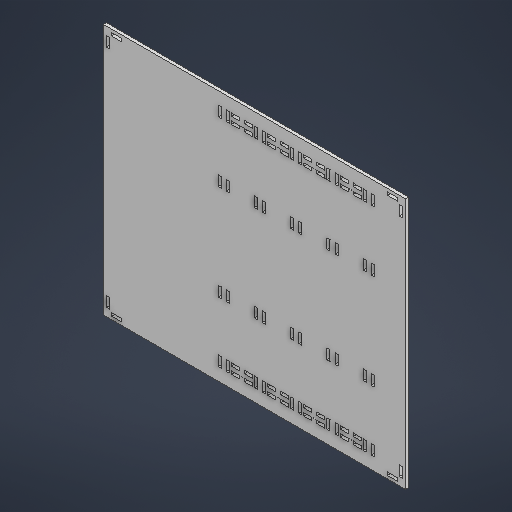
# Autodesk Inventor part: base_parqueo
Saved by Autodesk Inventor 2026 (Build 300175000, 175)
## iProperties
Created: 2026-05-15
Part Number: base_parqueo
Material: Generic
Document SubType Name: Modeling
Designer: juana
Density: 1 g/cm^3
Appearance: Default
Author: juana
Autodesk Inventor part; units mm, degrees
ref_plane "YZ Plane" through (0, 0, 0) normal (1, 0, 0) x (0, 1, 0)
ref_plane "XZ Plane" through (0, 0, 0) normal (0, 1, 0) x (-1, 0, 0)
ref_plane "XY Plane" through (0, 0, 0) normal (0, 0, 1) x (1, 0, 0)
sketch "Sketch1" plane through (0, 0, 0) normal (0, 0, 1) x (1, 0, 0)
  line L0 (300, -250) -> (0, -250)
  line L1 (0, -250) -> (0, 0)
  line L2 (0, 0) -> (300, 0)
  line L3 (300, 0) -> (300, -250)
  dimension "d0" = 250
  dimension "d1" = 300
  constraints: 8 end point, 2 coincident, 2 parallel, 1 horizontal, 1 horizontal alignment, 1 perpendicular, 1 vertical alignment
  measures "d0" distance of L2.end L0.start
  measures "d1" distance of L0.start L0.end
extrude "Extrusion1" add sketch "Sketch1" along normal blind 3
sketch "Sketch2" plane through (0, 0, 3) normal (0, 0, 1) x (1, 0, 0)
  line L0 (8, -247) -> (18, -247)
  line L1 (18, -247) -> (18, -244)
  line L2 (18, -244) -> (8, -244)
  line L3 (8, -244) -> (8, -247)
  line L4 (3, -242) -> (3, -232)
  line L5 (3, -232) -> (6, -232)
  line L6 (0, -250) -> (300, -250) construction
  line L7 (0, 0) -> (0, -250) construction
  line L8 (150, -250) -> (150, 0) construction
  line L9 (300, 0) -> (0, 0) construction
  line L10 (0, -125) -> (300, -125) construction
  line L11 (300, -250) -> (300, 0) construction
  line L12 (3, -242) -> (6, -242)
  line L13 (6, -242) -> (6, -232)
  line L14 (292, -247) -> (282, -247)
  line L15 (282, -247) -> (282, -244)
  line L16 (282, -244) -> (292, -244)
  line L17 (292, -244) -> (292, -247)
  line L18 (297, -242) -> (297, -232)
  line L19 (297, -232) -> (294, -232)
  line L20 (297, -242) -> (294, -242)
  line L21 (294, -242) -> (294, -232)
  line L22 (8, -3) -> (18, -3)
  line L23 (18, -3) -> (18, -6)
  line L24 (18, -6) -> (8, -6)
  line L25 (8, -6) -> (8, -3)
  line L26 (3, -8) -> (3, -18)
  line L27 (3, -18) -> (6, -18)
  line L28 (3, -8) -> (6, -8)
  line L29 (6, -8) -> (6, -18)
  line L30 (292, -3) -> (282, -3)
  line L31 (282, -6) -> (292, -6)
  line L32 (292, -6) -> (292, -3)
  line L33 (297, -8) -> (294, -8)
  line L34 (282, -3) -> (282, -6)
  line L35 (297, -8) -> (297, -18)
  line L36 (297, -18) -> (294, -18)
  line L37 (294, -8) -> (294, -18)
  point P0 (0, 0)
  point P1 (300, 0)
  dimension "d4" = 8
  dimension "d5" = 3
  dimension "d6" = 10
  dimension "d7" = 3
  dimension "d8" = 10
  dimension "d9" = 3
  dimension "d10" = 3
  dimension "d11" = 8
  constraints: 76 end point, 24 symmetric about line, 4 midpoint, 3 coincident, 3 horizontal, 2 parallel, 2 vertical, 1 perpendicular, 1 vertical alignment
  measures "d4" distance from line of L6.start L3
  measures "d5" distance from line of L6.start L0
  measures "d6" distance of L4.start L4.end
  measures "d7" distance of L2.end L0.start
  measures "d8" distance of L0.start L0.end
  measures "d9" distance of L4.start L12.end
  measures "d10" distance between parallel lines of L7 L4
  measures "d11" distance between parallel lines of L6 L12
extrude "Extrusion2" cut sketch "Sketch2" against normal blind 3
sketch "Sketch3" plane through (0, 0, 3) normal (0, 0, 1) x (1, 0, 0)
  line L0 (125, -12.5) -> (250, -12.5) construction
  line L1 (250, -12.5) -> (250, -237.5) construction
  line L2 (250, -237.5) -> (125, -237.5) construction
  line L3 (125, -237.5) -> (125, -12.5) construction
  line L4 (0, 0) -> (0, -250) construction
  line L5 (300, 0) -> (0, 0) construction
  line L6 (125, -12.5) -> (150, -12.5) construction
  line L7 (150, -12.5) -> (150, -82.5) construction
  line L8 (150, -82.5) -> (125, -82.5) construction
  line L9 (125, -82.5) -> (125, -12.5) construction
  line L10 (125, -12.5) -> (122, -12.5)
  line L11 (122, -12.5) -> (122, -22.5)
  line L12 (122, -22.5) -> (125, -22.5)
  line L13 (125, -22.5) -> (125, -12.5)
  line L14 (125, -82.5) -> (122, -82.5)
  line L15 (122, -82.5) -> (122, -72.5)
  line L16 (122, -72.5) -> (125, -72.5)
  line L17 (125, -72.5) -> (125, -82.5)
  line L18 (122, -72.5) -> (117, -72.5) construction
  line L19 (117, -72.5) -> (117, -82.5) construction
  line L20 (117, -82.5) -> (122, -82.5) construction
  line L21 (122, -82.5) -> (122, -72.5) construction
  line L22 (0, -125) -> (300, -125) construction
  line L23 (300, -250) -> (300, 0) construction
  line L24 (125, -47.5) -> (250, -47.5) construction
  line L25 (119.5, -72.5) -> (119.5, -82.5) construction
  line L26 (114, -82.5) -> (117, -82.5)
  line L27 (117, -82.5) -> (117, -72.5)
  line L28 (117, -72.5) -> (114, -72.5)
  line L29 (114, -72.5) -> (114, -82.5)
  line L30 (117, -82.5) -> (117, -72.5) construction
  line L31 (125, -12.5) -> (122, -12.5)
  line L32 (122, -12.5) -> (122, -22.5)
  line L33 (122, -22.5) -> (125, -22.5)
  line L34 (125, -22.5) -> (125, -12.5)
  line L35 (122, -22.5) -> (117, -22.5) construction
  line L36 (117, -22.5) -> (117, -12.5) construction
  line L37 (117, -12.5) -> (122, -12.5) construction
  line L38 (122, -12.5) -> (122, -22.5) construction
  line L39 (119.5, -22.5) -> (119.5, -12.5) construction
  line L40 (117, -22.5) -> (114, -22.5)
  line L41 (114, -22.5) -> (114, -12.5)
  line L42 (117, -12.5) -> (117, -22.5) construction
  line L43 (117, -12.5) -> (117, -22.5)
  line L44 (114, -12.5) -> (117, -12.5)
  line L45 (158, -22.5) -> (161, -22.5)
  line L46 (158, -22.5) -> (161, -22.5)
  line L47 (153, -22.5) -> (150, -22.5)
  line L48 (158, -22.5) -> (153, -22.5) construction
  line L49 (155.5, -22.5) -> (155.5, -12.5) construction
  line L50 (150, -12.5) -> (153, -12.5)
  line L51 (161, -12.5) -> (158, -12.5)
  line L52 (161, -12.5) -> (158, -12.5)
  line L53 (161, -22.5) -> (161, -12.5)
  line L54 (161, -22.5) -> (161, -12.5)
  line L55 (158, -12.5) -> (158, -22.5)
  line L56 (158, -12.5) -> (158, -22.5)
  line L57 (153, -22.5) -> (153, -12.5) construction
  line L58 (153, -12.5) -> (153, -22.5)
  line L59 (153, -12.5) -> (158, -12.5) construction
  line L60 (150, -22.5) -> (150, -12.5)
  line L61 (158, -12.5) -> (158, -22.5) construction
  line L62 (153, -12.5) -> (153, -22.5) construction
  line L63 (194, -22.5) -> (197, -22.5)
  line L64 (194, -22.5) -> (197, -22.5)
  line L65 (189, -22.5) -> (186, -22.5)
  line L66 (194, -22.5) -> (189, -22.5) construction
  line L67 (191.5, -22.5) -> (191.5, -12.5) construction
  line L68 (186, -12.5) -> (189, -12.5)
  line L69 (197, -12.5) -> (194, -12.5)
  line L70 (197, -12.5) -> (194, -12.5)
  line L71 (197, -22.5) -> (197, -12.5)
  line L72 (197, -22.5) -> (197, -12.5)
  line L73 (194, -12.5) -> (194, -22.5)
  line L74 (194, -12.5) -> (194, -22.5)
  line L75 (189, -22.5) -> (189, -12.5) construction
  line L76 (189, -12.5) -> (189, -22.5)
  line L77 (189, -12.5) -> (194, -12.5) construction
  line L78 (186, -22.5) -> (186, -12.5)
  line L79 (194, -12.5) -> (194, -22.5) construction
  line L80 (189, -12.5) -> (189, -22.5) construction
  line L81 (230, -22.5) -> (233, -22.5)
  line L82 (230, -22.5) -> (233, -22.5)
  line L83 (225, -22.5) -> (222, -22.5)
  line L84 (230, -22.5) -> (225, -22.5) construction
  line L85 (227.5, -22.5) -> (227.5, -12.5) construction
  line L86 (222, -12.5) -> (225, -12.5)
  line L87 (233, -12.5) -> (230, -12.5)
  line L88 (233, -12.5) -> (230, -12.5)
  line L89 (233, -22.5) -> (233, -12.5)
  line L90 (233, -22.5) -> (233, -12.5)
  line L91 (230, -12.5) -> (230, -22.5)
  line L92 (230, -12.5) -> (230, -22.5)
  line L93 (225, -22.5) -> (225, -12.5) construction
  line L94 (225, -12.5) -> (225, -22.5)
  line L95 (225, -12.5) -> (230, -12.5) construction
  line L96 (222, -22.5) -> (222, -12.5)
  line L97 (230, -12.5) -> (230, -22.5) construction
  line L98 (225, -12.5) -> (225, -22.5) construction
  line L99 (266, -22.5) -> (269, -22.5)
  line L100 (266, -22.5) -> (269, -22.5)
  line L101 (261, -22.5) -> (258, -22.5)
  line L102 (266, -22.5) -> (261, -22.5) construction
  line L103 (263.5, -22.5) -> (263.5, -12.5) construction
  line L104 (258, -12.5) -> (261, -12.5)
  line L105 (269, -12.5) -> (266, -12.5)
  line L106 (269, -12.5) -> (266, -12.5)
  line L107 (269, -22.5) -> (269, -12.5)
  line L108 (269, -22.5) -> (269, -12.5)
  line L109 (266, -12.5) -> (266, -22.5)
  line L110 (266, -12.5) -> (266, -22.5)
  line L111 (261, -22.5) -> (261, -12.5) construction
  line L112 (261, -12.5) -> (261, -22.5)
  line L113 (261, -12.5) -> (266, -12.5) construction
  line L114 (258, -22.5) -> (258, -12.5)
  line L115 (266, -12.5) -> (266, -22.5) construction
  line L116 (261, -12.5) -> (261, -22.5) construction
  line L117 (125, -82.5) -> (250, -82.5) construction
  line L118 (158, -72.5) -> (161, -72.5)
  line L119 (158, -72.5) -> (161, -72.5)
  line L120 (153, -72.5) -> (150, -72.5)
  line L121 (158, -72.5) -> (153, -72.5) construction
  line L122 (155.5, -72.5) -> (155.5, -82.5) construction
  line L123 (150, -82.5) -> (153, -82.5)
  line L124 (161, -82.5) -> (158, -82.5)
  line L125 (161, -82.5) -> (158, -82.5)
  line L126 (161, -72.5) -> (161, -82.5)
  line L127 (161, -72.5) -> (161, -82.5)
  line L128 (158, -82.5) -> (158, -72.5)
  line L129 (158, -82.5) -> (158, -72.5)
  line L130 (153, -72.5) -> (153, -82.5) construction
  line L131 (153, -82.5) -> (153, -72.5)
  line L132 (153, -82.5) -> (158, -82.5) construction
  line L133 (150, -72.5) -> (150, -82.5)
  line L134 (158, -82.5) -> (158, -72.5) construction
  line L135 (153, -82.5) -> (153, -72.5) construction
  line L136 (194, -72.5) -> (197, -72.5)
  line L137 (194, -72.5) -> (197, -72.5)
  line L138 (189, -72.5) -> (186, -72.5)
  line L139 (194, -72.5) -> (189, -72.5) construction
  line L140 (191.5, -72.5) -> (191.5, -82.5) construction
  line L141 (186, -82.5) -> (189, -82.5)
  line L142 (197, -82.5) -> (194, -82.5)
  line L143 (197, -82.5) -> (194, -82.5)
  line L144 (197, -72.5) -> (197, -82.5)
  line L145 (197, -72.5) -> (197, -82.5)
  line L146 (194, -82.5) -> (194, -72.5)
  line L147 (194, -82.5) -> (194, -72.5)
  line L148 (189, -72.5) -> (189, -82.5) construction
  line L149 (189, -82.5) -> (189, -72.5)
  line L150 (189, -82.5) -> (194, -82.5) construction
  line L151 (186, -72.5) -> (186, -82.5)
  line L152 (194, -82.5) -> (194, -72.5) construction
  line L153 (189, -82.5) -> (189, -72.5) construction
  line L154 (230, -72.5) -> (233, -72.5)
  line L155 (230, -72.5) -> (233, -72.5)
  line L156 (225, -72.5) -> (222, -72.5)
  line L157 (230, -72.5) -> (225, -72.5) construction
  line L158 (227.5, -72.5) -> (227.5, -82.5) construction
  line L159 (222, -82.5) -> (225, -82.5)
  line L160 (233, -82.5) -> (230, -82.5)
  line L161 (233, -82.5) -> (230, -82.5)
  line L162 (233, -72.5) -> (233, -82.5)
  line L163 (233, -72.5) -> (233, -82.5)
  line L164 (230, -82.5) -> (230, -72.5)
  line L165 (230, -82.5) -> (230, -72.5)
  line L166 (225, -72.5) -> (225, -82.5) construction
  line L167 (225, -82.5) -> (225, -72.5)
  line L168 (225, -82.5) -> (230, -82.5) construction
  line L169 (222, -72.5) -> (222, -82.5)
  line L170 (230, -82.5) -> (230, -72.5) construction
  line L171 (225, -82.5) -> (225, -72.5) construction
  line L172 (266, -72.5) -> (269, -72.5)
  line L173 (266, -72.5) -> (269, -72.5)
  line L174 (261, -72.5) -> (258, -72.5)
  line L175 (266, -72.5) -> (261, -72.5) construction
  line L176 (263.5, -72.5) -> (263.5, -82.5) construction
  line L177 (258, -82.5) -> (261, -82.5)
  line L178 (269, -82.5) -> (266, -82.5)
  line L179 (269, -82.5) -> (266, -82.5)
  line L180 (269, -72.5) -> (269, -82.5)
  line L181 (269, -72.5) -> (269, -82.5)
  line L182 (266, -82.5) -> (266, -72.5)
  line L183 (266, -82.5) -> (266, -72.5)
  line L184 (261, -72.5) -> (261, -82.5) construction
  line L185 (261, -82.5) -> (261, -72.5)
  line L186 (261, -82.5) -> (266, -82.5) construction
  line L187 (258, -72.5) -> (258, -82.5)
  line L188 (266, -82.5) -> (266, -72.5) construction
  line L189 (261, -82.5) -> (261, -72.5) construction
  line L190 (125, -237.5) -> (250, -237.5) construction
  line L191 (125, -237.5) -> (150, -237.5) construction
  line L192 (150, -237.5) -> (150, -167.5) construction
  line L193 (150, -167.5) -> (125, -167.5) construction
  line L194 (125, -167.5) -> (125, -237.5) construction
  line L195 (125, -237.5) -> (122, -237.5)
  line L196 (122, -237.5) -> (122, -227.5)
  line L197 (122, -227.5) -> (125, -227.5)
  line L198 (125, -227.5) -> (125, -237.5)
  line L199 (125, -167.5) -> (122, -167.5)
  line L200 (122, -167.5) -> (122, -177.5)
  line L201 (122, -177.5) -> (125, -177.5)
  line L202 (125, -177.5) -> (125, -167.5)
  line L203 (122, -177.5) -> (117, -177.5) construction
  line L204 (117, -177.5) -> (117, -167.5) construction
  line L205 (117, -167.5) -> (122, -167.5) construction
  line L206 (122, -167.5) -> (122, -177.5) construction
  line L207 (125, -202.5) -> (250, -202.5) construction
  line L208 (119.5, -177.5) -> (119.5, -167.5) construction
  line L209 (117, -177.5) -> (114, -177.5)
  line L210 (114, -177.5) -> (114, -167.5)
  line L211 (117, -167.5) -> (117, -177.5) construction
  line L212 (117, -167.5) -> (117, -177.5)
  line L213 (114, -167.5) -> (117, -167.5)
  line L214 (117, -227.5) -> (117, -237.5) construction
  line L215 (117, -237.5) -> (117, -227.5)
  line L216 (119.5, -227.5) -> (119.5, -237.5) construction
  line L217 (122, -237.5) -> (122, -227.5) construction
  line L218 (122, -237.5) -> (122, -227.5)
  line L219 (125, -227.5) -> (125, -237.5)
  line L220 (125, -237.5) -> (122, -237.5)
  line L221 (114, -237.5) -> (117, -237.5)
  line L222 (114, -227.5) -> (114, -237.5)
  line L223 (117, -237.5) -> (117, -227.5) construction
  line L224 (122, -227.5) -> (117, -227.5) construction
  line L225 (122, -227.5) -> (125, -227.5)
  line L226 (117, -227.5) -> (114, -227.5)
  line L227 (117, -237.5) -> (122, -237.5) construction
  line L228 (158, -227.5) -> (161, -227.5)
  line L229 (158, -227.5) -> (161, -227.5)
  line L230 (153, -227.5) -> (150, -227.5)
  line L231 (158, -227.5) -> (153, -227.5) construction
  line L232 (155.5, -227.5) -> (155.5, -237.5) construction
  line L233 (150, -237.5) -> (153, -237.5)
  line L234 (161, -237.5) -> (158, -237.5)
  line L235 (161, -237.5) -> (158, -237.5)
  line L236 (161, -227.5) -> (161, -237.5)
  line L237 (161, -227.5) -> (161, -237.5)
  line L238 (158, -237.5) -> (158, -227.5)
  line L239 (158, -237.5) -> (158, -227.5)
  line L240 (153, -227.5) -> (153, -237.5) construction
  line L241 (153, -237.5) -> (153, -227.5)
  line L242 (153, -237.5) -> (158, -237.5) construction
  line L243 (150, -227.5) -> (150, -237.5)
  line L244 (158, -237.5) -> (158, -227.5) construction
  line L245 (153, -237.5) -> (153, -227.5) construction
  line L246 (194, -227.5) -> (197, -227.5)
  line L247 (194, -227.5) -> (197, -227.5)
  line L248 (189, -227.5) -> (186, -227.5)
  line L249 (194, -227.5) -> (189, -227.5) construction
  line L250 (191.5, -227.5) -> (191.5, -237.5) construction
  line L251 (186, -237.5) -> (189, -237.5)
  line L252 (197, -237.5) -> (194, -237.5)
  line L253 (197, -237.5) -> (194, -237.5)
  line L254 (197, -227.5) -> (197, -237.5)
  line L255 (197, -227.5) -> (197, -237.5)
  line L256 (194, -237.5) -> (194, -227.5)
  line L257 (194, -237.5) -> (194, -227.5)
  line L258 (189, -227.5) -> (189, -237.5) construction
  line L259 (189, -237.5) -> (189, -227.5)
  line L260 (189, -237.5) -> (194, -237.5) construction
  line L261 (186, -227.5) -> (186, -237.5)
  line L262 (194, -237.5) -> (194, -227.5) construction
  line L263 (189, -237.5) -> (189, -227.5) construction
  line L264 (230, -227.5) -> (233, -227.5)
  line L265 (230, -227.5) -> (233, -227.5)
  line L266 (225, -227.5) -> (222, -227.5)
  line L267 (230, -227.5) -> (225, -227.5) construction
  line L268 (227.5, -227.5) -> (227.5, -237.5) construction
  line L269 (222, -237.5) -> (225, -237.5)
  line L270 (233, -237.5) -> (230, -237.5)
  line L271 (233, -237.5) -> (230, -237.5)
  line L272 (233, -227.5) -> (233, -237.5)
  line L273 (233, -227.5) -> (233, -237.5)
  line L274 (230, -237.5) -> (230, -227.5)
  line L275 (230, -237.5) -> (230, -227.5)
  line L276 (225, -227.5) -> (225, -237.5) construction
  line L277 (225, -237.5) -> (225, -227.5)
  line L278 (225, -237.5) -> (230, -237.5) construction
  line L279 (222, -227.5) -> (222, -237.5)
  line L280 (230, -237.5) -> (230, -227.5) construction
  line L281 (225, -237.5) -> (225, -227.5) construction
  line L282 (266, -227.5) -> (269, -227.5)
  line L283 (266, -227.5) -> (269, -227.5)
  line L284 (261, -227.5) -> (258, -227.5)
  line L285 (266, -227.5) -> (261, -227.5) construction
  line L286 (263.5, -227.5) -> (263.5, -237.5) construction
  line L287 (258, -237.5) -> (261, -237.5)
  line L288 (269, -237.5) -> (266, -237.5)
  line L289 (269, -237.5) -> (266, -237.5)
  line L290 (269, -227.5) -> (269, -237.5)
  line L291 (269, -227.5) -> (269, -237.5)
  line L292 (266, -237.5) -> (266, -227.5)
  line L293 (266, -237.5) -> (266, -227.5)
  line L294 (261, -227.5) -> (261, -237.5) construction
  line L295 (261, -237.5) -> (261, -227.5)
  line L296 (261, -237.5) -> (266, -237.5) construction
  line L297 (258, -227.5) -> (258, -237.5)
  line L298 (266, -237.5) -> (266, -227.5) construction
  line L299 (261, -237.5) -> (261, -227.5) construction
  line L300 (158, -177.5) -> (161, -177.5)
  line L301 (158, -177.5) -> (161, -177.5)
  line L302 (150, -177.5) -> (150, -167.5)
  line L303 (150, -167.5) -> (153, -167.5)
  line L304 (153, -177.5) -> (150, -177.5)
  line L305 (153, -167.5) -> (153, -177.5) construction
  line L306 (153, -177.5) -> (153, -167.5) construction
  line L307 (153, -167.5) -> (153, -177.5)
  line L308 (153, -167.5) -> (158, -167.5) construction
  line L309 (158, -177.5) -> (153, -177.5) construction
  line L310 (158, -167.5) -> (158, -177.5)
  line L311 (158, -167.5) -> (158, -177.5) construction
  line L312 (158, -167.5) -> (158, -177.5)
  line L313 (161, -167.5) -> (158, -167.5)
  line L314 (161, -167.5) -> (158, -167.5)
  line L315 (161, -177.5) -> (161, -167.5)
  line L316 (161, -177.5) -> (161, -167.5)
  line L317 (155.5, -177.5) -> (155.5, -167.5) construction
  line L318 (125, -167.5) -> (250, -167.5) construction
  line L319 (186, -177.5) -> (186, -167.5)
  line L320 (186, -167.5) -> (189, -167.5)
  line L321 (189, -177.5) -> (186, -177.5)
  line L322 (189, -167.5) -> (189, -177.5) construction
  line L323 (189, -177.5) -> (189, -167.5) construction
  line L324 (189, -167.5) -> (189, -177.5)
  line L325 (191.5, -177.5) -> (191.5, -167.5) construction
  line L326 (189, -167.5) -> (194, -167.5) construction
  line L327 (194, -177.5) -> (189, -177.5) construction
  line L328 (194, -167.5) -> (194, -177.5)
  line L329 (194, -167.5) -> (194, -177.5)
  line L330 (194, -177.5) -> (197, -177.5)
  line L331 (194, -177.5) -> (197, -177.5)
  line L332 (197, -167.5) -> (194, -167.5)
  line L333 (197, -167.5) -> (194, -167.5)
  line L334 (197, -177.5) -> (197, -167.5)
  line L335 (197, -177.5) -> (197, -167.5)
  line L336 (194, -167.5) -> (194, -177.5) construction
  line L337 (222, -177.5) -> (222, -167.5)
  line L338 (222, -167.5) -> (225, -167.5)
  line L339 (225, -177.5) -> (222, -177.5)
  line L340 (225, -177.5) -> (225, -167.5) construction
  line L341 (225, -167.5) -> (225, -177.5)
  line L342 (225, -167.5) -> (225, -177.5) construction
  line L343 (227.5, -177.5) -> (227.5, -167.5) construction
  line L344 (225, -167.5) -> (230, -167.5) construction
  line L345 (230, -177.5) -> (225, -177.5) construction
  line L346 (230, -167.5) -> (230, -177.5)
  line L347 (230, -167.5) -> (230, -177.5) construction
  line L348 (230, -167.5) -> (230, -177.5)
  line L349 (233, -177.5) -> (233, -167.5)
  line L350 (233, -177.5) -> (233, -167.5)
  line L351 (230, -177.5) -> (233, -177.5)
  line L352 (230, -177.5) -> (233, -177.5)
  line L353 (233, -167.5) -> (230, -167.5)
  line L354 (233, -167.5) -> (230, -167.5)
  line L355 (261, -167.5) -> (261, -177.5) construction
  line L356 (261, -177.5) -> (261, -167.5) construction
  line L357 (261, -167.5) -> (261, -177.5)
  line L358 (266, -177.5) -> (261, -177.5) construction
  line L359 (266, -167.5) -> (266, -177.5)
  line L360 (266, -167.5) -> (266, -177.5) construction
  line L361 (266, -167.5) -> (266, -177.5)
  line L362 (266, -177.5) -> (269, -177.5)
  line L363 (266, -177.5) -> (269, -177.5)
  line L364 (263.5, -177.5) -> (263.5, -167.5) construction
  line L365 (261, -177.5) -> (258, -177.5)
  line L366 (258, -177.5) -> (258, -167.5)
  line L367 (269, -177.5) -> (269, -167.5)
  line L368 (269, -177.5) -> (269, -167.5)
  line L369 (269, -167.5) -> (266, -167.5)
  line L370 (269, -167.5) -> (266, -167.5)
  line L371 (261, -167.5) -> (266, -167.5) construction
  line L372 (258, -167.5) -> (261, -167.5)
  point P0 (125, -125)
  point P1 (187.5, -12.5)
  point P2 (187.5, -82.5)
  point P3 (150, -82.5)
  point P4 (187.5, -237.5)
  point P5 (150, -167.5)
  point P6 (187.5, -167.5)
  dimension "d14" = 25
  dimension "d15" = 70
  dimension "d16" = 125
  dimension "d17" = 225
  dimension "d18" = 3
  dimension "d19" = 10
  dimension "d20" = 3
  dimension "d21" = 10
  dimension "d22" = 5
  dimension "d25" = 36
  dimension "d30" = 125
  constraints: 740 end point, 235 symmetric about line, 10 parallel, 7 horizontal, 7 midpoint, 5 perpendicular, 2 horizontal alignment, 1 coincident, 1 point on line, 1 vertical alignment, 132 other
  measures "d14" distance of L6.start L6.end
  measures "d15" distance of L6.end L7.end
  measures "d16" distance of L0.start L0.end
  measures "d17" distance of L2.end L0.start
  measures "d18" distance of L6.start L10.end
  measures "d19" distance of L10.end L11.end
  measures "d20" distance of L8.end L14.end
  measures "d21" distance of L14.end L15.end
  measures "d22" distance of L15.end L18.end
  measures "d25" distance of L0.start L52.start
  measures "d30" distance between parallel lines of L4 L3
extrude "Extrusion3" cut sketch "Sketch3" against normal blind 3
sketch "Sketch4" plane through (0, 0, 3) normal (0, 0, 1) x (1, 0, 0)
  line L0 (114, -12.5) -> (114, -22.5) construction
  line L1 (266, -237.5) -> (269, -237.5) construction
  line L2 (114, -12.5) -> (269, -12.5) construction
  line L3 (269, -12.5) -> (269, -237.5) construction
  line L4 (269, -237.5) -> (114, -237.5) construction
  line L5 (114, -237.5) -> (114, -12.5) construction
  line L6 (114, -167.5) -> (117, -167.5) construction
  line L7 (125, -177.5) -> (125, -167.5) construction
  line L8 (114, -167.5) -> (125, -167.5) construction
  line L9 (125, -167.5) -> (125, -177.5) construction
  line L10 (125, -177.5) -> (114, -177.5) construction
  line L11 (114, -177.5) -> (114, -167.5) construction
  line L12 (114, -227.5) -> (125, -227.5) construction
  line L13 (125, -227.5) -> (125, -237.5) construction
  line L14 (125, -237.5) -> (114, -237.5) construction
  line L15 (114, -237.5) -> (114, -227.5) construction
  line L16 (127, -227.5) -> (135, -227.5)
  line L17 (135, -227.5) -> (135, -230.5)
  line L18 (135, -230.5) -> (127, -230.5)
  line L19 (127, -230.5) -> (127, -227.5)
  line L20 (114, -227.5) -> (161, -227.5) construction
  line L21 (161, -227.5) -> (161, -237.5) construction
  line L22 (161, -237.5) -> (114, -237.5) construction
  line L23 (114, -237.5) -> (114, -227.5) construction
  line L24 (137.5, -227.5) -> (137.5, -237.5) construction
  line L25 (148, -227.5) -> (140, -227.5)
  line L26 (140, -227.5) -> (140, -230.5)
  line L27 (140, -230.5) -> (148, -230.5)
  line L28 (148, -230.5) -> (148, -227.5)
  circle A0 centre (137.5, -230.65) radius 0.15
  circle A1 centre (138.5, -230.65) radius 0.15
  circle A2 centre (136.5, -230.65) radius 0.15
  line L29 (140, -230.5) -> (134.9519, -230.5) construction
  line L30 (125, -232.5) -> (150, -232.5) construction
  line L31 (150, -227.5) -> (150, -237.5) construction
  line L32 (127, -237.5) -> (135, -237.5)
  line L33 (135, -237.5) -> (135, -234.5)
  line L34 (135, -234.5) -> (127, -234.5)
  line L35 (127, -234.5) -> (127, -237.5)
  line L36 (148, -237.5) -> (140, -237.5)
  line L37 (140, -237.5) -> (140, -234.5)
  line L38 (140, -234.5) -> (148, -234.5)
  line L39 (148, -234.5) -> (148, -237.5)
  circle A3 centre (137.5, -234.35) radius 0.15
  circle A4 centre (138.5, -234.35) radius 0.15
  circle A5 centre (136.5, -234.35) radius 0.15
  line L40 (140, -234.5) -> (134.9519, -234.5) construction
  line L41 (171, -230.5) -> (163, -230.5)
  line L42 (171, -227.5) -> (171, -230.5)
  line L43 (176, -230.5) -> (170.9519, -230.5) construction
  circle A6 centre (172.5, -230.65) radius 0.15
  circle A7 centre (173.5, -230.65) radius 0.15
  circle A8 centre (174.5, -230.65) radius 0.15
  circle A9 centre (172.5, -234.35) radius 0.15
  circle A10 centre (173.5, -234.35) radius 0.15
  circle A11 centre (174.5, -234.35) radius 0.15
  line L44 (173.5, -227.5) -> (173.5, -237.5) construction
  line L45 (163, -237.5) -> (171, -237.5)
  line L46 (171, -237.5) -> (171, -234.5)
  line L47 (171, -234.5) -> (163, -234.5)
  line L48 (163, -227.5) -> (171, -227.5)
  line L49 (163, -234.5) -> (163, -237.5)
  line L50 (176, -234.5) -> (170.9519, -234.5) construction
  line L51 (163, -230.5) -> (163, -227.5)
  line L52 (184, -227.5) -> (176, -227.5)
  line L53 (176, -227.5) -> (176, -230.5)
  line L54 (176, -230.5) -> (184, -230.5)
  line L55 (184, -230.5) -> (184, -227.5)
  line L56 (176, -237.5) -> (176, -234.5)
  line L57 (184, -237.5) -> (176, -237.5)
  line L58 (176, -234.5) -> (184, -234.5)
  line L59 (184, -234.5) -> (184, -237.5)
  line L60 (207, -230.5) -> (199, -230.5)
  line L61 (207, -227.5) -> (207, -230.5)
  line L62 (212, -230.5) -> (206.9519, -230.5) construction
  circle A12 centre (208.5, -230.65) radius 0.15
  circle A13 centre (209.5, -230.65) radius 0.15
  circle A14 centre (210.5, -230.65) radius 0.15
  circle A15 centre (208.5, -234.35) radius 0.15
  circle A16 centre (209.5, -234.35) radius 0.15
  circle A17 centre (210.5, -234.35) radius 0.15
  line L63 (209.5, -227.5) -> (209.5, -237.5) construction
  line L64 (199, -237.5) -> (207, -237.5)
  line L65 (207, -237.5) -> (207, -234.5)
  line L66 (207, -234.5) -> (199, -234.5)
  line L67 (199, -227.5) -> (207, -227.5)
  line L68 (199, -234.5) -> (199, -237.5)
  line L69 (212, -234.5) -> (206.9519, -234.5) construction
  line L70 (199, -230.5) -> (199, -227.5)
  line L71 (220, -227.5) -> (212, -227.5)
  line L72 (212, -227.5) -> (212, -230.5)
  line L73 (212, -230.5) -> (220, -230.5)
  line L74 (220, -230.5) -> (220, -227.5)
  line L75 (212, -237.5) -> (212, -234.5)
  line L76 (220, -237.5) -> (212, -237.5)
  line L77 (212, -234.5) -> (220, -234.5)
  line L78 (220, -234.5) -> (220, -237.5)
  line L79 (243, -230.5) -> (235, -230.5)
  line L80 (243, -227.5) -> (243, -230.5)
  line L81 (248, -230.5) -> (242.9519, -230.5) construction
  circle A18 centre (244.5, -230.65) radius 0.15
  circle A19 centre (245.5, -230.65) radius 0.15
  circle A20 centre (246.5, -230.65) radius 0.15
  circle A21 centre (244.5, -234.35) radius 0.15
  circle A22 centre (245.5, -234.35) radius 0.15
  circle A23 centre (246.5, -234.35) radius 0.15
  line L82 (245.5, -227.5) -> (245.5, -237.5) construction
  line L83 (235, -237.5) -> (243, -237.5)
  line L84 (243, -237.5) -> (243, -234.5)
  line L85 (243, -234.5) -> (235, -234.5)
  line L86 (235, -227.5) -> (243, -227.5)
  line L87 (235, -234.5) -> (235, -237.5)
  line L88 (248, -234.5) -> (242.9519, -234.5) construction
  line L89 (235, -230.5) -> (235, -227.5)
  line L90 (256, -227.5) -> (248, -227.5)
  line L91 (248, -227.5) -> (248, -230.5)
  line L92 (248, -230.5) -> (256, -230.5)
  line L93 (256, -230.5) -> (256, -227.5)
  line L94 (248, -237.5) -> (248, -234.5)
  line L95 (256, -237.5) -> (248, -237.5)
  line L96 (248, -234.5) -> (256, -234.5)
  line L97 (256, -234.5) -> (256, -237.5)
  line L98 (114, -167.5) -> (269, -167.5) construction
  line L99 (269, -167.5) -> (269, -237.5) construction
  line L100 (269, -237.5) -> (114, -237.5) construction
  line L101 (114, -237.5) -> (114, -167.5) construction
  line L102 (114, -202.5) -> (269, -202.5) construction
  line L103 (114, -125) -> (269, -125) construction
  line L104 (127, -22.5) -> (135, -22.5)
  line L105 (135, -22.5) -> (135, -19.5)
  line L106 (135, -19.5) -> (127, -19.5)
  line L107 (127, -19.5) -> (127, -22.5)
  line L108 (137.5, -22.5) -> (137.5, -12.5) construction
  line L109 (148, -22.5) -> (140, -22.5)
  line L110 (140, -22.5) -> (140, -19.5)
  line L111 (140, -19.5) -> (148, -19.5)
  line L112 (148, -19.5) -> (148, -22.5)
  circle A24 centre (137.5, -19.35) radius 0.15
  circle A25 centre (138.5, -19.35) radius 0.15
  circle A26 centre (136.5, -19.35) radius 0.15
  line L113 (140, -19.5) -> (134.9519, -19.5) construction
  line L114 (127, -12.5) -> (135, -12.5)
  line L115 (127, -15.5) -> (127, -12.5)
  line L116 (135, -15.5) -> (127, -15.5)
  line L117 (140, -15.5) -> (134.9519, -15.5) construction
  circle A27 centre (136.5, -15.65) radius 0.15
  circle A28 centre (137.5, -15.65) radius 0.15
  circle A29 centre (138.5, -15.65) radius 0.15
  line L118 (135, -12.5) -> (135, -15.5)
  line L119 (140, -12.5) -> (140, -15.5)
  line L120 (148, -12.5) -> (140, -12.5)
  line L121 (140, -15.5) -> (148, -15.5)
  line L122 (148, -15.5) -> (148, -12.5)
  line L123 (171, -19.5) -> (163, -19.5)
  line L124 (171, -22.5) -> (171, -19.5)
  line L125 (176, -19.5) -> (170.9519, -19.5) construction
  circle A30 centre (172.5, -19.35) radius 0.15
  circle A31 centre (173.5, -19.35) radius 0.15
  circle A32 centre (174.5, -19.35) radius 0.15
  circle A33 centre (172.5, -15.65) radius 0.15
  circle A34 centre (173.5, -15.65) radius 0.15
  circle A35 centre (174.5, -15.65) radius 0.15
  line L126 (173.5, -22.5) -> (173.5, -12.5) construction
  line L127 (163, -12.5) -> (171, -12.5)
  line L128 (171, -12.5) -> (171, -15.5)
  line L129 (171, -15.5) -> (163, -15.5)
  line L130 (163, -22.5) -> (171, -22.5)
  line L131 (163, -15.5) -> (163, -12.5)
  line L132 (176, -15.5) -> (170.9519, -15.5) construction
  line L133 (163, -19.5) -> (163, -22.5)
  line L134 (184, -22.5) -> (176, -22.5)
  line L135 (176, -22.5) -> (176, -19.5)
  line L136 (176, -19.5) -> (184, -19.5)
  line L137 (184, -19.5) -> (184, -22.5)
  line L138 (176, -12.5) -> (176, -15.5)
  line L139 (184, -12.5) -> (176, -12.5)
  line L140 (176, -15.5) -> (184, -15.5)
  line L141 (184, -15.5) -> (184, -12.5)
  line L142 (207, -19.5) -> (199, -19.5)
  line L143 (207, -22.5) -> (207, -19.5)
  line L144 (212, -19.5) -> (206.9519, -19.5) construction
  circle A36 centre (208.5, -19.35) radius 0.15
  circle A37 centre (209.5, -19.35) radius 0.15
  circle A38 centre (210.5, -19.35) radius 0.15
  circle A39 centre (208.5, -15.65) radius 0.15
  circle A40 centre (209.5, -15.65) radius 0.15
  circle A41 centre (210.5, -15.65) radius 0.15
  line L145 (209.5, -22.5) -> (209.5, -12.5) construction
  line L146 (199, -12.5) -> (207, -12.5)
  line L147 (207, -12.5) -> (207, -15.5)
  line L148 (207, -15.5) -> (199, -15.5)
  line L149 (199, -22.5) -> (207, -22.5)
  line L150 (199, -15.5) -> (199, -12.5)
  line L151 (212, -15.5) -> (206.9519, -15.5) construction
  line L152 (199, -19.5) -> (199, -22.5)
  line L153 (220, -22.5) -> (212, -22.5)
  line L154 (212, -22.5) -> (212, -19.5)
  line L155 (212, -19.5) -> (220, -19.5)
  line L156 (220, -19.5) -> (220, -22.5)
  line L157 (212, -12.5) -> (212, -15.5)
  line L158 (220, -12.5) -> (212, -12.5)
  line L159 (212, -15.5) -> (220, -15.5)
  line L160 (220, -15.5) -> (220, -12.5)
  line L161 (243, -19.5) -> (235, -19.5)
  line L162 (243, -22.5) -> (243, -19.5)
  line L163 (248, -19.5) -> (242.9519, -19.5) construction
  circle A42 centre (244.5, -19.35) radius 0.15
  circle A43 centre (245.5, -19.35) radius 0.15
  circle A44 centre (246.5, -19.35) radius 0.15
  circle A45 centre (244.5, -15.65) radius 0.15
  circle A46 centre (245.5, -15.65) radius 0.15
  circle A47 centre (246.5, -15.65) radius 0.15
  line L164 (245.5, -22.5) -> (245.5, -12.5) construction
  line L165 (235, -12.5) -> (243, -12.5)
  line L166 (243, -12.5) -> (243, -15.5)
  line L167 (243, -15.5) -> (235, -15.5)
  line L168 (235, -22.5) -> (243, -22.5)
  line L169 (235, -15.5) -> (235, -12.5)
  line L170 (248, -15.5) -> (242.9519, -15.5) construction
  line L171 (235, -19.5) -> (235, -22.5)
  line L172 (256, -22.5) -> (248, -22.5)
  line L173 (248, -22.5) -> (248, -19.5)
  line L174 (248, -19.5) -> (256, -19.5)
  line L175 (256, -19.5) -> (256, -22.5)
  line L176 (248, -12.5) -> (248, -15.5)
  line L177 (256, -12.5) -> (248, -12.5)
  line L178 (248, -15.5) -> (256, -15.5)
  line L179 (256, -15.5) -> (256, -12.5)
  point P0 (0, 0)
  point P1 (117, -227.5)
  dimension "d33" = 3
  dimension "d34" = 8
  dimension "d35" = 2
  dimension "d36" = 0.3
  dimension "d37" = 1
  dimension "d38" = 1
  dimension "d41" = 36
  constraints: 350 end point, 120 symmetric about line, 48 centre point, 27 point on line, 12 parallel, 8 midpoint, 7 horizontal, 6 perpendicular, 4 horizontal alignment, 2 equal radius, 1 coincident, 1 tangent, 180 other
  measures "d33" distance of L16.end L17.end
  measures "d34" distance of L16.start L16.end
  measures "d35" distance between parallel lines of L13 L19
  measures "d36" diameter of A1
  measures "d37" distance of A1.centre A0.centre
  measures "d38" distance of A0.centre A2.centre
  measures "d41" distance of L29.end L43.end
extrude "Extrusion4" cut sketch "Sketch4" against normal blind 36 contours L16 L17 L18 L19 | L28 L27 L26 L25 | L35 L34 L33 L32 | L36 L37 L38 L39 | A3 | A4 | A5 | L41 L51 L48 L42 | A9 | A10 | A11 | L49 L47 L46 L45 | L55 L54 L53 L52 | L56 L58 L59 L57 | L60 L70 L67 L61 | A15 | A16 | A17 | L68 L66 L65 L64 | L74 L73 L72 L71 | L75 L77 L78 L76 | L79 L89 L86 L80 | A21 | A22 | A23 | L87 L85 L84 L83 | L93 L92 L91 L90 | L94 L96 L97 L95 | L107 L106 L105 L104 | L109 L110 L111 L112 | A24 | A25 | A26 | L114 L118 L116 L115 | L120 L122 L121 L119 | L124 L130 L133 L123 | A30 | A31 | A32 | L127 L128 L129 L131 | L134 L135 L136 L137 | L139 L141 L140 L138 | L143 L149 L152 L142 | A36 | A37 | A38 | L146 L147 L148 L150 | L153 L154 L155 L156 | L158 L160 L159 L157 | L162 L168 L171 L161 | A42 | A43 | A44 | L165 L166 L167 L169 | L172 L173 L174 L175 | L177 L179 L178 L176
equation "\"d46\" = d41"
body "Solid1"
